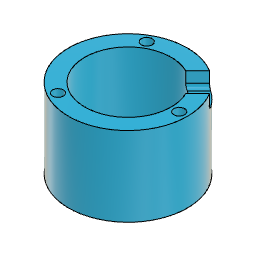
entretoise_moteur_KOSMOS3-0 (Autodesk Fusion 360 design; units mm, degrees)
Autodesk Fusion 360 part; units mm, degrees
sketch "Esquisse1" plane through (0, 0, 0) normal (0, 0, 1) x (1, 0, 0)
  circle A0 centre (0, 0) radius 22
  circle A1 centre (0, 0) radius 16
  circle A2 centre (19, 0) radius 2
  circle A3 centre (-9.5, 16.4545) radius 2
  circle A4 centre (-9.5, -16.4545) radius 2
  dimension "d1" = 44
  dimension "d2" = 32
  dimension "d3" = 4
  dimension "d4" = 19
  dimension "d6" = 360
  constraint coincident A0.centre A1.centre
  measures "d1" diameter of A0
  measures "d2" diameter of A1
  measures "d3" diameter of A2
  measures "d4" distance of A0.centre A2.centre
extrude "Extrusion1" add sketch "Esquisse1" along normal blind 29.45
ref_plane "Plan de construction1" through (0, 0, 12.125) normal (0.707107, 0.707107, 0) x (0, 0, 1)
sketch "Esquisse5" plane through (0, 0, 12.125) normal (0.707107, 0.707107, 0) x (0, 0, 1)
  line L0 (11.825, 0) -> (11.825, -5.2)
  line L1 (11.825, -5.2) -> (17.325, -5.2)
  line L2 (17.325, -5.2) -> (17.325, 0)
  circle A0 through (17.325, 16, 0) (17.325, -8, 13.8564) (17.325, -8, -13.8564)
  line L3 (11.825, 0) -> (11.825, 5.2)
  line L4 (11.825, 5.2) -> (17.325, 5.2)
  line L5 (17.325, 5.2) -> (11.825, 5.2)
  line L6 (11.825, 5.2) -> (11.825, -5.2)
  line L7 (11.825, -5.2) -> (17.325, -5.2)
  line L8 (17.325, -5.2) -> (17.325, 5.2)
  dimension "d22" = 5.2
  dimension "d23" = 5.5
  dimension "d24" = 5.5
  dimension "d25" = 5.2
  constraint vertical L0
  constraint horizontal L1
  constraint vertical L2
  constraint vertical L3
  constraint horizontal L4
  constraint horizontal L5
  constraint vertical L6
  constraint horizontal L7
  constraint vertical L8
  measures "d22" distance of L0.start L0.end
  measures "d23" distance of L0.end L1.end
  measures "d24" distance of L3.end L4.end
  measures "d25" distance of L0.start L3.end
extrude "Extrusion3" cut sketch "Esquisse5" along normal blind 22
fillet "Congé1" radius 1.5 2 edges at (9.2306, 16.5845, 23.95) (16.5845, 9.2306, 23.95)
sketch "Esquisse3" plane through (0, 0, 0) normal (1, 0, 0) x (0, 1, 0)
  line L0 (-5, 32) -> (5, 32)
  line L1 (5, 32) -> (5, 28)
  line L2 (4, 27) -> (-4, 27)
  line L3 (-5, 28) -> (-5, 32)
  arc A0 (-5, 28) -> (-4, 27) centre (-4, 28) ccw
  arc A1 (4, 27) -> (5, 28) centre (4, 28) ccw
  point P0 (5, 27)
  point P1 (-5, 27)
  dimension "d10" = 5
  dimension "d11" = 10
  dimension "d12" = 1
  dimension "d13" = 1
  constraint horizontal L0
  constraint vertical L1
  constraint horizontal L2
  constraint vertical L3
  constraint coincident P1 L3
  constraint coincident P1 L2
  constraint tangent L3 A0
  constraint tangent L2 A0
  constraint coincident P0 L2
  constraint coincident P0 L1
  constraint tangent L2 A1
  constraint tangent L1 A1
  measures "d10" distance of L0.start P1
  measures "d11" distance of P0 P1
  measures "d12" radius of A0
  measures "d13" radius of A1
